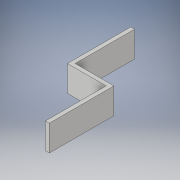
# Autodesk Inventor part: recreat1
Saved by Autodesk Inventor 2019 (Build 230136000, 136)
## iProperties
Created: 2021-10-25
Part Number: recreat1
Material: 一般
Document SubType Name: Modeling
Designer: yuta
Density: 1 g/cm^3
Appearance: 既定
Author: yuta
Autodesk Inventor part; units mm, degrees
ref_plane "YZ Plane" through (0, 0, 0) normal (1, 0, 0) x (0, 1, 0)
ref_plane "XZ Plane" through (0, 0, 0) normal (0, 1, 0) x (-1, 0, 0)
ref_plane "XY Plane" through (0, 0, 0) normal (0, 0, 1) x (1, 0, 0)
sketch "スケッチ1" plane through (0, 0, 0) normal (0, 1, 0) x (-1, 0, 0)
  line L0 (1.7293, 44.1636) -> (-1.2707, 44.1636)
  line L1 (-1.2707, 44.1636) -> (-1.2707, -5.8364)
  line L2 (-1.2707, -5.8364) -> (1.7293, -5.8364)
  line L3 (1.7293, -5.8364) -> (1.7293, 44.1636)
  line L4 (31.7293, -2.8364) -> (1.7293, -2.8364)
  line L5 (1.7293, -2.8364) -> (1.7293, -5.8364)
  line L6 (1.7293, -5.8364) -> (31.7293, -5.8364)
  line L7 (31.7293, -5.8364) -> (31.7293, -2.8364)
  line L8 (31.7293, -5.8364) -> (28.7293, -5.8364)
  line L9 (28.7293, -5.8364) -> (28.7293, -51.7922)
  line L10 (28.7293, -51.7922) -> (31.7293, -51.7922)
  line L11 (31.7293, -51.7922) -> (31.7293, -5.8364)
  point P0 (0, 0)
  dimension "d0" = 3
  dimension "d1" = 50
  dimension "d2" = 30
  dimension "d3" = 3
  dimension "d4" = 3
  constraints: 24 end point, 6 parallel, 4 collinear, 3 horizontal, 3 perpendicular
  measures "d0" distance of L2.end L1.end
  measures "d1" distance of L0.end L1.end
  measures "d2" distance of L6.end L5.end
  measures "d3" distance of L6.end L4.start
  measures "d4" distance of L10.end L9.end
extrude "押し出し1" add sketch "スケッチ1" along normal blind 20
